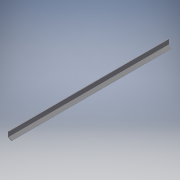
# Autodesk Inventor part: gurnee_top
Saved by Autodesk Inventor 2018 (Build 220112000, 112)
## iProperties
Created: 2018-05-02
Part Number: gurnee_top
Material: 一般
Document SubType Name: Modeling
Designer: ku_sk
Density: 1 g/cm^3
Appearance: 既定
Author: ku_sk
Autodesk Inventor part; units mm, degrees
ref_plane "YZ Plane" through (0, 0, 0) normal (1, 0, 0) x (0, 1, 0)
ref_plane "XZ Plane" through (0, 0, 0) normal (0, 1, 0) x (-1, 0, 0)
ref_plane "XY Plane" through (0, 0, 0) normal (0, 0, 1) x (1, 0, 0)
sketch "スケッチ1" plane through (0, 0, 0) normal (0, 1, 0) x (-1, 0, 0)
  line L0 (0, 0) -> (0, 7)
  line L1 (0, 7) -> (1, 7)
  line L2 (1, 7) -> (1, -0.5774)
  line L3 (1, -0.5774) -> (-4.1962, -3.5774)
  line L4 (-4.1962, -3.5774) -> (-4.6962, -2.7113)
  line L5 (-4.6962, -2.7113) -> (0, 0)
  dimension "d0" = 7
  dimension "d1" = 1
  dimension "d2" = 1
  dimension "d5" = 120
  dimension "d6" = 6
  constraints: 12 end point, 3 perpendicular, 1 parallel, 1 vertical
  measures "d0" distance of L0.start L0.end
  measures "d1" distance of L0.end L1.end
  measures "d2" distance of L3.end L4.end
  measures "d5" angle of L5 L0
  measures "d6" distance of L2.end L3.end
extrude "押し出し1" add sketch "スケッチ1" along normal mid plane 245
